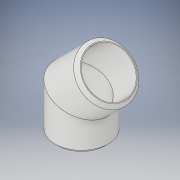
# Autodesk Inventor part: Elbow 45degrees 1.25IN D
Saved by Autodesk Inventor 2019 (Build 230136000, 136)
## iProperties
Created: 2019-07-05
Part Number: Elbow 45degrees 1.25IN D
Material: PVC-Piping
Document SubType Name: Modeling
Designer: J. LENDI
Mass: 55.2594 g
Surface Area: 214.15 cm^2
Volume: 39.471 cm^3
Density: 1.4 g/cm^3
Appearance: Smooth - White
Author: J. LENDI
Autodesk Inventor part; units mm, degrees
ref_plane "YZ Plane" through (0, 0, 0) normal (1, 0, 0) x (0, 1, 0)
ref_plane "XZ Plane" through (0, 0, 0) normal (0, 1, 0) x (-1, 0, 0)
ref_plane "XY Plane" through (0, 0, 0) normal (0, 0, 1) x (1, 0, 0)
sketch "Sketch1" plane through (0, 0, 0) normal (0, 1, 0) x (-1, 0, 0)
  circle A0 centre (0, 0) radius 25.0063
  circle A1 centre (0, 0) radius 21.082
  dimension "d0" = 50.0126
  dimension "d1" = 42.164
  constraints: 2 centre point, 2 coincident
  measures "d0" diameter of A0
  measures "d1" diameter of A1
sketch "Sketch2" plane through (0, 0, 0) normal (0, 0, 1) x (1, 0, 0)
  line L0 (0, 0) -> (0, 36.068)
  line L1 (0, 36.068) -> (25.5039, 61.5719)
  line L2 (0, 36.068) -> (0, 32.2314) construction
  line L3 (-35.1083, 0) -> (35.606, 0) construction
  line L4 (25.0063, 0) -> (-25.0063, 0) construction
  dimension "d2" = 45
  dimension "d12" = 25.5039
  dimension "d13" = 36.068
  dimension "d14" = 61.5719
  constraints: 6 end point, 2 vertical
  measures "d2" angle of L1 L2
  measures "d12" horizontal distance of L0.end L1.end
  measures "d13" distance of L0.start L0.end
  measures "d14" distance from line of L3 L1.end
sweep "Sweep1" add profiles "Sketch1" path "Sketch2"
chamfer "Chamfer1" distance 3.175 angle 45 2 edges at (43.1861, 43.8898, 0) (25.0063, 0, 0)
equation "\"d12\" = 0.707107 * d13"
body "Solid1"
